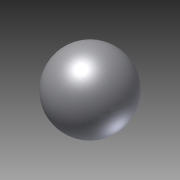
# Autodesk Inventor part: Ball
Saved by Autodesk Inventor 2012 SP2 (Build 160219200, 219)
## iProperties
Created: 2013-08-24
Part Number: Ball
Material: Default
Document SubType Name: Modeling
Designer: 1
Density: 1 g/cm^3
Author: 1
Autodesk Inventor part; units mm, degrees
ref_plane "YZ Plane" through (0, 0, 0) normal (1, 0, 0) x (0, 1, 0)
ref_plane "XZ Plane" through (0, 0, 0) normal (0, 1, 0) x (-1, 0, 0)
ref_plane "XY Plane" through (0, 0, 0) normal (0, 0, 1) x (1, 0, 0)
sketch "Sketch1" plane through (0, 0, 0) normal (0, 0, 1) x (1, 0, 0)
  arc A0 (0, 9.398) -> (0, -9.398) centre (0, 0) ccw
  line L0 (0, 9.398) -> (0, -9.398) construction
  line L1 (0, 9.398) -> (0, -9.398)
  dimension "d1" = 9.398
  constraints: 4 end point, 3 point on circle, 1 centre point, 1 coincident, 1 collinear
  measures "d1" radius of A0
revolve "Revolution1" add sketch "Sketch1" angle 360 about axis through (0, 9.398, 0) along (0, -1, 0)
body "Solid1"
